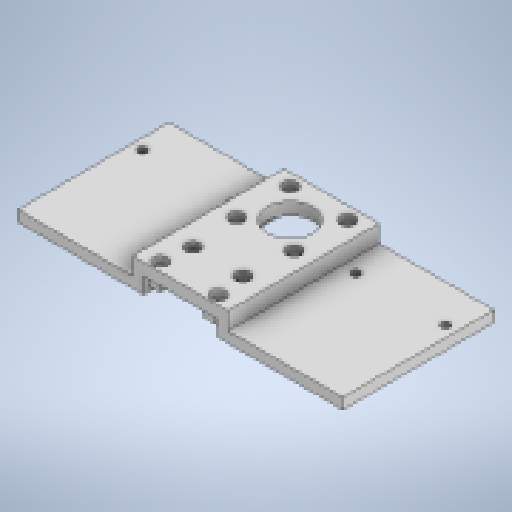
# Autodesk Inventor part: gripper_fixer
Saved by Autodesk Inventor 2024 (Build 280153000, 153)
## iProperties
Created: 2023-09-15
Part Number: gripper_fixer
Material: Generic
Document SubType Name: Modeling
Designer: 박동준
Density: 1 g/cm^3
Appearance: Default
Author: 박동준
Autodesk Inventor part; units mm, degrees
ref_plane "YZ Plane" through (0, 0, 0) normal (1, 0, 0) x (0, 1, 0)
ref_plane "XZ Plane" through (0, 0, 0) normal (0, 1, 0) x (-1, 0, 0)
ref_plane "XY Plane" through (0, 0, 0) normal (0, 0, 1) x (1, 0, 0)
sketch "Sketch1" plane through (0, 0, 0) normal (0, 0, 1) x (1, 0, 0)
  line L0 (-13.245, 7.83) -> (-13.245, 3)
  line L1 (-13.245, 3) -> (-45.245, 3)
  line L2 (-45.245, 3) -> (-45.245, 0)
  line L3 (-45.245, 0) -> (-10.245, 0)
  line L4 (-10.245, 0) -> (-10.245, 4.43)
  line L5 (-10.245, 4.43) -> (10.245, 4.43)
  line L6 (10.245, 4.43) -> (10.245, 0)
  line L7 (10.245, 0) -> (45.245, 0)
  line L8 (45.245, 0) -> (45.245, 3)
  line L9 (45.245, 3) -> (13.245, 3)
  line L10 (13.245, 3) -> (13.245, 7.83)
  line L11 (13.245, 7.83) -> (-13.245, 7.83)
  line L12 (-10.245, 0) -> (10.245, 0) construction
  point P0 (0, 0)
  point P1 (0, 7.83)
  point P2 (0, 0)
  point P3 (-13.245, 5.415)
  dimension "d0" = 20.49
  dimension "d1" = 3.4
  dimension "d3" = 1.43
  dimension "d4" = 3
  dimension "d5" = 3
  dimension "d6" = 35
  dimension "d7" = 35
  dimension "d9" = 13.245
  dimension "d10" = 3
  constraints: 26 end point, 9 perpendicular, 3 midpoint, 2 point on line, 2 vertical, 1 collinear, 1 horizontal alignment, 1 vertical alignment
  measures "d0" distance between parallel lines of L6 L4
  measures "d1" distance between parallel lines of L11 L5
  measures "d3" distance between parallel lines of L9 L5
  measures "d4" distance of L7.end L8.end
  measures "d5" distance of L1.end L2.end
  measures "d6" distance of L6.end L7.end
  measures "d7" distance of L2.end L3.end
  measures "d9" distance from line of L0 point (0, 7.83)
  measures "d10" distance from line of point (-13.245, 5.415) L4
extrude "Extrusion1" add sketch "Sketch1" along normal mid plane 41.1
sketch "Sketch3" plane through (-13.245, 7.83, 20.55) normal (0, 1, 0) x (1, 0, 0)
  circle A0 centre (13.245, 3.18) radius 0.7835 projected
  circle A1 centre (6.245, 10.48) radius 0.7835 projected
  circle A2 centre (20.245, 10.48) radius 0.7835 projected
  circle A3 centre (5.245, 23.7) radius 0.7835 projected
  circle A4 centre (21.245, 23.7) radius 0.7835 projected
  line L0 (19.315, 1.78) -> (7.175, 1.78) projected
  line L1 (19.315, 1.78) -> (19.315, 2.5) projected
  arc A5 (21.315, 4.5) -> (19.315, 2.5) centre (21.315, 2.5) ccw projected
  line L2 (21.315, 4.5) -> (22.035, 4.5) projected
  line L3 (22.035, 36.6) -> (22.035, 4.5) projected
  line L4 (22.035, 36.6) -> (21.315, 36.6) projected
  arc A6 (19.315, 38.6) -> (21.315, 36.6) centre (21.315, 38.6) ccw projected
  line L5 (19.315, 38.6) -> (19.315, 39.32) projected
  line L6 (7.175, 39.32) -> (19.315, 39.32) projected
  line L7 (7.175, 39.32) -> (7.175, 38.6) projected
  arc A7 (5.175, 36.6) -> (7.175, 38.6) centre (5.175, 38.6) ccw projected
  line L8 (5.175, 36.6) -> (4.455, 36.6) projected
  line L9 (4.455, 4.5) -> (4.455, 36.6) projected
  line L10 (4.455, 4.5) -> (5.175, 4.5) projected
  arc A8 (7.175, 2.5) -> (5.175, 4.5) centre (5.175, 2.5) ccw projected
  line L11 (7.175, 2.5) -> (7.175, 1.78) projected
  circle A9 centre (13.245, 30.6) radius 6.4 projected
  point P0 (13.245, 20.55)
hole "Hole1" at (7, 7.83, 10.07) at (8, 7.83, -3.15) at (-8, 7.83, -3.15) at (-7, 7.83, 10.07) direction (0, -1, 0) diameter 2.1 end through all counterbore diameter 4 counterbore depth 2
sketch "Sketch4" plane through (-13.245, 7.83, 20.55) normal (0, 1, 0) x (1, 0, 0)
  circle A0 centre (13.245, 3.18) radius 0.7835 projected
  circle A1 centre (6.245, 10.48) radius 0.7835 projected
  circle A2 centre (20.245, 10.48) radius 0.7835 projected
  circle A3 centre (5.245, 23.7) radius 0.7835 projected
  circle A4 centre (21.245, 23.7) radius 0.7835 projected
  line L0 (19.315, 1.78) -> (7.175, 1.78) projected
  line L1 (19.315, 1.78) -> (19.315, 2.5) projected
  arc A5 (21.315, 4.5) -> (19.315, 2.5) centre (21.315, 2.5) ccw projected
  line L2 (21.315, 4.5) -> (22.035, 4.5) projected
  line L3 (22.035, 36.6) -> (22.035, 4.5) projected
  line L4 (22.035, 36.6) -> (21.315, 36.6) projected
  arc A6 (19.315, 38.6) -> (21.315, 36.6) centre (21.315, 38.6) ccw projected
  line L5 (19.315, 38.6) -> (19.315, 39.32) projected
  line L6 (7.175, 39.32) -> (19.315, 39.32) projected
  line L7 (7.175, 39.32) -> (7.175, 38.6) projected
  arc A7 (5.175, 36.6) -> (7.175, 38.6) centre (5.175, 38.6) ccw projected
  line L8 (5.175, 36.6) -> (4.455, 36.6) projected
  line L9 (4.455, 4.5) -> (4.455, 36.6) projected
  line L10 (4.455, 4.5) -> (5.175, 4.5) projected
  arc A8 (7.175, 2.5) -> (5.175, 4.5) centre (5.175, 2.5) ccw projected
  line L11 (7.175, 2.5) -> (7.175, 1.78) projected
  circle A9 centre (13.245, 30.6) radius 6.4 projected
  circle A10 centre (13.245, 30.6) radius 6.5
  point P0 (13.245, 20.55)
  dimension "d28" = 13
  constraints: 1 centre point, 1 coincident
  measures "d28" diameter of A10
extrude "Extrusion2" cut sketch "Sketch4" against normal up to surface (3.4 mm away) contours A9
sketch "Sketch6" plane through (-10.245, 4.43, 20.55) normal (0, -1, 0) x (1, 0, 0)
  arc A0 (19.315, -40.6) -> (20.315, -39.6) centre (19.315, -39.6) ccw projected
  line L0 (16.315, -40.6) -> (19.315, -40.6) projected
  line L1 (16.315, -38.6) -> (16.315, -40.6) projected
  arc A1 (18.315, -36.6) -> (16.315, -38.6) centre (18.315, -38.6) ccw projected
  line L2 (20.315, -36.6) -> (18.315, -36.6) projected
  line L3 (20.315, -39.6) -> (20.315, -36.6) projected
  circle A2 centre (18.315, -38.6) radius 0.7835 projected
  circle A3 centre (2.175, -38.6) radius 0.7835 projected
  arc A4 (0.175, -39.6) -> (1.175, -40.6) centre (1.175, -39.6) ccw projected
  line L4 (0.175, -36.6) -> (0.175, -39.6) projected
  line L5 (2.175, -36.6) -> (0.175, -36.6) projected
  arc A5 (4.175, -38.6) -> (2.175, -36.6) centre (2.175, -38.6) ccw projected
  line L6 (4.175, -40.6) -> (4.175, -38.6) projected
  line L7 (1.175, -40.6) -> (4.175, -40.6) projected
  circle A6 centre (18.315, -2.5) radius 0.7835 projected
  arc A7 (20.315, -1.5) -> (19.315, -0.5) centre (19.315, -1.5) ccw projected
  line L8 (20.315, -4.5) -> (20.315, -1.5) projected
  line L9 (18.315, -4.5) -> (20.315, -4.5) projected
  arc A8 (16.315, -2.5) -> (18.315, -4.5) centre (18.315, -2.5) ccw projected
  line L10 (16.315, -0.5) -> (16.315, -2.5) projected
  line L11 (19.315, -0.5) -> (16.315, -0.5) projected
  arc A9 (1.175, -0.5) -> (0.175, -1.5) centre (1.175, -1.5) ccw projected
  line L12 (4.175, -0.5) -> (1.175, -0.5) projected
  line L13 (4.175, -2.5) -> (4.175, -0.5) projected
  arc A10 (2.175, -4.5) -> (4.175, -2.5) centre (2.175, -2.5) ccw projected
  line L14 (0.175, -4.5) -> (2.175, -4.5) projected
  line L15 (0.175, -1.5) -> (0.175, -4.5) projected
  circle A11 centre (2.175, -2.5) radius 0.7835 projected
  circle A12 centre (10.245, -30.6) radius 6.4 projected
  circle A13 centre (3.245, -10.48) radius 1.05 projected
  circle A14 centre (2.245, -23.7) radius 1.05 projected
  circle A15 centre (18.245, -23.7) radius 1.05 projected
  circle A16 centre (17.245, -10.48) radius 1.05 projected
  line L16 (20.49, -41.1) -> (20.49, 0) projected
  line L17 (0, 0) -> (20.49, 0) projected
  line L18 (0, -41.1) -> (0, 0) projected
  line L19 (20.49, -41.1) -> (0, -41.1) projected
  line L20 (20.315, -0.5) -> (20.49, -0.5)
  line L21 (0.175, -41.1) -> (0, -41.1)
  circle A17 centre (2.075, -2.4) radius 0.7835
  arc A18 (2.075, -4.4) -> (4.075, -2.4) centre (2.075, -2.4) ccw
  line L22 (2.075, -4.4) -> (0, -4.4)
  line L23 (0, -4.4) -> (0, 0)
  line L24 (0, 0) -> (4.075, 0)
  line L25 (4.075, 0) -> (4.075, -2.4)
  line L26 (10.245, -40.6) -> (10.245, 0.4051) construction
  line L27 (0, -20.55) -> (20.49, -20.55) construction
  line L28 (20.49, -41.1) -> (20.49, 0)
  circle A19 centre (18.415, -2.4) radius 0.7835
  arc A20 (16.415, -2.4) -> (18.415, -4.4) centre (18.415, -2.4) ccw
  line L29 (18.415, -4.4) -> (20.49, -4.4)
  line L30 (20.49, 0) -> (16.415, 0)
  line L31 (16.415, 0) -> (16.415, -2.4)
  line L32 (20.49, 0) -> (20.49, -41.1)
  line L33 (0, -41.1) -> (20.49, -41.1)
  line L34 (0, 0) -> (0, -41.1)
  circle A21 centre (2.075, -38.7) radius 0.7835
  arc A22 (4.075, -38.7) -> (2.075, -36.7) centre (2.075, -38.7) ccw
  line L35 (2.075, -36.7) -> (0, -36.7)
  line L36 (4.075, -41.1) -> (4.075, -38.7)
  line L37 (18.415, -36.7) -> (20.49, -36.7)
  arc A23 (18.415, -36.7) -> (16.415, -38.7) centre (18.415, -38.7) ccw
  line L38 (16.415, -41.1) -> (16.415, -38.7)
  circle A24 centre (18.415, -38.7) radius 0.7835
  point P0 (10.245, -20.55)
  point P1 (0.175, -0.5)
  point P2 (0, -36.6)
  point P3 (20.49, -36.6)
  point P4 (20.49, -4.5)
  point P5 (0, -4.5)
  point P6 (19.315, -0.5)
  point P7 (4.175, 0)
  point P8 (16.315, 0)
  point P9 (16.315, -41.1)
  point P10 (4.175, -41.1)
  point P11 (4.075, -0.5)
  point P12 (0.175, -4.4)
  point P13 (20.315, -4.4)
  point P14 (16.415, -0.5)
  point P15 (0.175, -36.7)
  point P16 (4.075, -41.1)
  point P17 (4.075, -40.6)
  point P18 (16.415, -40.6)
  point P19 (20.315, -36.7)
  dimension "d54" = 1.567
  dimension "d55" = 2.075
  dimension "d56" = 2.4
  dimension "d57" = 2
  dimension "d58" = 2
  dimension "d59" = 2
  constraints: 38 end point, 22 symmetric about line, 18 point on line, 8 centre point, 8 point on circle, 4 coincident, 4 perpendicular, 2 midpoint, 1 collinear, 6 other
  measures "d54" diameter of A17
  measures "d55" distance from line of L18 A17.centre
  measures "d56" distance from line of L17 A17.centre
  measures "d57" radius of A18
  measures "d58" distance from line of L25 A17.centre
  measures "d59" distance from line of L22 A17.centre
extrude "Extrusion3" add sketch "Sketch6" along normal blind 2 contours L0 L38 A23 L37 L3 A0 | A0 L3 L37 L16 L19 L38 L0 | L19 L18 L35 L4 A4 L7 L36 | L29 L8 A7 L11 L31 L17 L16 | L7 A4 L4 L35 A22 L36 | L29 A20 L31 L11 A7 L8 | L18 L17 L25 L12 A9 L15 L22 | L15 A9 L12 L25 A18 L22 | A2 A24 | A2 A24 | A24 A2 | A3 A21 | A21 A3 | A3 A21 | A6 A19 | A6 A19 | A19 A6 | A11 A17 | A17 A11 | A11 A17
sketch "Sketch7" plane through (-13.245, 7.83, 20.55) normal (0, 1, 0) x (1, 0, 0)
  circle A0 centre (13.245, 3.18) radius 0.7835 projected
  circle A1 centre (6.245, 10.48) radius 0.7835 projected
  circle A2 centre (20.245, 10.48) radius 0.7835 projected
  circle A3 centre (5.245, 23.7) radius 0.7835 projected
  circle A4 centre (21.245, 23.7) radius 0.7835 projected
  line L0 (19.315, 1.78) -> (7.175, 1.78) projected
  line L1 (19.315, 1.78) -> (19.315, 2.5) projected
  arc A5 (21.315, 4.5) -> (19.315, 2.5) centre (21.315, 2.5) ccw projected
  line L2 (21.315, 4.5) -> (22.035, 4.5) projected
  line L3 (22.035, 36.6) -> (22.035, 4.5) projected
  line L4 (22.035, 36.6) -> (21.315, 36.6) projected
  arc A6 (19.315, 38.6) -> (21.315, 36.6) centre (21.315, 38.6) ccw projected
  line L5 (19.315, 38.6) -> (19.315, 39.32) projected
  line L6 (7.175, 39.32) -> (19.315, 39.32) projected
  line L7 (7.175, 39.32) -> (7.175, 38.6) projected
  arc A7 (5.175, 36.6) -> (7.175, 38.6) centre (5.175, 38.6) ccw projected
  line L8 (5.175, 36.6) -> (4.455, 36.6) projected
  line L9 (4.455, 4.5) -> (4.455, 36.6) projected
  line L10 (4.455, 4.5) -> (5.175, 4.5) projected
  arc A8 (7.175, 2.5) -> (5.175, 4.5) centre (5.175, 2.5) ccw projected
  line L11 (7.175, 2.5) -> (7.175, 1.78) projected
  circle A9 centre (13.245, 30.6) radius 6.4 projected
  point P0 (13.245, 20.55)
hole "Hole2" at (8.07, 7.83, -18.05) at (-8.07, 7.83, -18.05) at (-8.07, 7.83, 18.05) at (8.07, 7.83, 18.05) direction (0, -1, 0) diameter 2.1 end through all counterbore diameter 4 counterbore depth 2
sketch "Sketch8" plane through (13.245, 3, 20.55) normal (0, 1, 0) x (1, 0, 0)
  line L0 (0, 41.1) -> (0, 0)
  line L1 (32, 0) -> (0, 0) projected
  line L2 (32, 41.1) -> (32, 0) projected
  line L3 (0, 41.1) -> (32, 41.1) projected
  line L4 (-58.49, 41.1) -> (-58.49, 0) projected
  line L5 (-26.49, 0) -> (-58.49, 0) projected
  line L6 (-26.49, 0) -> (-26.49, 41.1) projected
  line L7 (-58.49, 41.1) -> (-26.49, 41.1) projected
  line L8 (32, 41.1) -> (32, 0) projected
  circle A0 centre (-13.245, 30.6) radius 6.4 projected
  line L9 (-13.245, 41) -> (-13.245, 0) construction
  point P0 (-13.245, 20.55)
  point P1 (-55.49, 30.65)
  point P2 (-30.49, 30.65)
  point P3 (-58.49, 20.55)
  point P4 (29, 30.65)
  point P5 (4, 30.65)
  dimension "d42" = 3
  dimension "d43" = 25
  dimension "d51" = 10.45
  dimension "d53" = 3
  constraints: 4 end point, 2 symmetric about line, 1 horizontal alignment, 1 midpoint, 1 vertical
  measures "d42" distance from line of L4 point (-55.49, 30.65)
  measures "d43" distance of point (-30.49, 30.65) point (-55.49, 30.65)
  measures "d51" distance from line of point (-30.49, 30.65) L7
  measures "d53" distance from line of L2 point (29, 30.65)
hole "Hole3" at (-42.245, 3, -10.1) at (-17.245, 3, -10.1) at (17.245, 3, -10.1) at (42.245, 3, -10.1) direction (0, -1, 0) diameter 2.459 end through all thread size "M3x0.5" class "6H" standard "ISO Metric profile"
body "Solid1"
